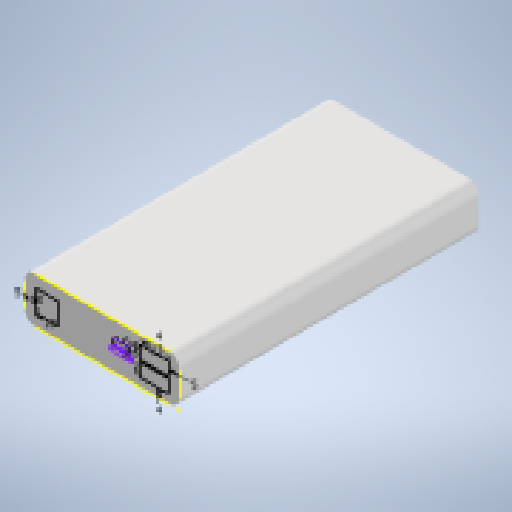
# Autodesk Inventor part: power bank
Saved by Autodesk Inventor 2023 (Build 270158000, 158)
## iProperties
Created: 2023-04-11
Part Number: power bank
Material: Generic
Document SubType Name: Modeling
Designer: ASARe-DAQ-PC
Density: 1 g/cm^3
Appearance: Default
Author: ASARe-DAQ-PC
Autodesk Inventor part; units mm, degrees
ref_plane "YZ Plane" through (0, 0, 0) normal (1, 0, 0) x (0, 1, 0)
ref_plane "XZ Plane" through (0, 0, 0) normal (0, 1, 0) x (-1, 0, 0)
ref_plane "XY Plane" through (0, 0, 0) normal (0, 0, 1) x (1, 0, 0)
sketch "Sketch1" plane through (0, 0, 0) normal (0, 1, 0) x (-1, 0, 0)
  line L0 (0, 0) -> (71, 0)
  line L1 (71, 0) -> (71, -137)
  line L2 (71, -137) -> (0, -137)
  line L3 (0, -137) -> (0, 0)
  dimension "d0" = 137
  dimension "d1" = 71
  constraints: 8 end point, 2 parallel, 1 horizontal, 1 perpendicular
  measures "d0" distance of L2.end L0.start
  measures "d1" distance of L0.start L0.end
extrude "Extrusion1" add sketch "Sketch1" along normal blind 21
fillet "Fillet1" radius 5 4 edges at (0, 21, -68.5) (0, 0, -68.5) (-71, 21, -68.5) (-71, 0, -68.5)
sketch "Sketch2" plane through (-66, 0, 0) normal (0, 0, 1) x (1, 0, 0)
  line L0 (0, 15.5) -> (10, 15.5)
  line L1 (10, 15.5) -> (10, 5.5)
  line L2 (10, 5.5) -> (0, 5.5)
  line L3 (0, 5.5) -> (0, 15.5)
  line L4 (48, 17) -> (61, 17)
  line L5 (61, 17) -> (61, 11)
  line L6 (61, 11) -> (48, 11)
  line L7 (48, 11) -> (48, 17)
  line L8 (48, 10) -> (61, 10)
  line L9 (61, 10) -> (61, 4)
  line L10 (61, 4) -> (48, 4)
  line L11 (48, 4) -> (48, 10)
  line L12 (66, 5) -> (66, 16) projected
  line L13 (0, 0) -> (61, 0) projected
  line L14 (0, 21) -> (61, 21) projected
  line L15 (-5, 5) -> (-5, 16) projected
  line L16 (35.4, 13.6) -> (43, 13.6)
  line L17 (43, 13.6) -> (43, 11)
  line L18 (43, 11) -> (35.4, 11)
  line L19 (35.4, 11) -> (35.4, 13.6)
  line L20 (36.2, 10) -> (42.2, 10)
  line L21 (43.7, 8.5) -> (43.7, 8.3)
  line L22 (42.2, 6.8) -> (36.2, 6.8)
  line L23 (34.7, 8.3) -> (34.7, 8.5)
  arc A0 (36.2, 10) -> (34.7, 8.5) centre (36.2, 8.5) ccw
  arc A1 (43.7, 8.5) -> (42.2, 10) centre (42.2, 8.5) ccw
  arc A2 (34.7, 8.3) -> (36.2, 6.8) centre (36.2, 8.3) ccw
  arc A3 (42.2, 6.8) -> (43.7, 8.3) centre (42.2, 8.3) ccw
  line L24 (35.4, 12) -> (36.4, 11)
  line L25 (43, 12) -> (42, 11)
  point P0 (66, 0)
  point P1 (0, 10.5)
  point P2 (-5, 10.5)
  point P3 (43.7, 6.8)
  point P4 (34.7, 6.8)
  point P5 (39.2, 11)
  point P6 (39.2, 10)
  dimension "d5" = 6
  dimension "d6" = 6
  dimension "d7" = 13
  dimension "d8" = 5
  dimension "d9" = 4
  dimension "d10" = 4
  dimension "d11" = 5
  dimension "d12" = 10
  dimension "d13" = 10
  dimension "d14" = 7.6
  dimension "d15" = 2.6
  dimension "d16" = 5
  dimension "d17" = 3.2
  dimension "d19" = 9
  dimension "d20" = 1
  dimension "d21" = 1.5
  dimension "d26" = 45
  dimension "d27" = 45
  dimension "d28" = 1
  dimension "d29" = 1
  constraints: 44 end point, 10 parallel, 10 point on line, 8 point on circle, 8 tangent, 5 horizontal, 5 perpendicular, 4 centre point, 4 midpoint, 3 equal radius, 2 horizontal alignment, 1 vertical alignment
  measures "d5" distance of L6.end L4.start
  measures "d6" distance of L10.end L8.start
  measures "d7" distance of L4.start L4.end
  measures "d8" distance between parallel lines of L12 L5
  measures "d9" distance between parallel lines of L13 L10
  measures "d10" distance between parallel lines of L14 L4
  measures "d11" distance between parallel lines of L3 L15
  measures "d12" distance of L2.end L0.start
  measures "d13" distance of L1.end L2.end
  measures "d14" distance of L16.start L16.end
  measures "d15" distance of L16.end L17.end
  measures "d16" distance between parallel lines of L7 L17
  measures "d17" distance between parallel lines of L22 L20
  measures "d19" distance of point (43.7, 6.8) point (34.7, 6.8)
  measures "d20" distance between parallel lines of L20 L18
  measures "d21" radius of A0
  measures "d26" angle of L18 L24
  measures "d27" angle of L18 L25
  measures "d28" distance of L18.end L24.start
  measures "d29" distance of L17.end L25.start
extrude "Extrusion2" cut sketch "Sketch2" against normal blind 20 contours L4 L5 L6 L7 | L8 L9 L10 L11 | L16 L17 L25 L18 L24 L19 | L20 A1 L21 A3 L22 A2 L23 A0
extrude "Extrusion3" add sketch "Sketch2" along normal blind 1 contours L0 L1 L2 L3
sketch "Sketch3" plane through (-66, 0, 1) normal (0, 0, 1) x (1, 0, 0)
  circle A0 centre (5, 10.5) radius 3 construction
  arc A1 (3.0716, 12.7981) -> (6.9284, 12.7981) centre (5, 10.5) ccw
  line L0 (3.0716, 12.7981) -> (5, 10.5) construction
  line L1 (5, 10.5) -> (6.9284, 12.7981) construction
  line L2 (5, 10.5) -> (5, 13.5) construction
  line L3 (10, 5.5) -> (10, 15.5) projected
  line L4 (10, 15.5) -> (0, 15.5) projected
  circle A2 centre (5, 10.5) radius 2.5 construction
  arc A3 (3.393, 12.4151) -> (6.607, 12.4151) centre (5, 10.5) ccw
  arc A4 (3.393, 12.4151) -> (3.0716, 12.7981) centre (3.2323, 12.6066) ccw
  arc A5 (6.9284, 12.7981) -> (6.607, 12.4151) centre (6.7677, 12.6066) ccw
  line L5 (4.75, 14) -> (5.25, 14) construction
  line L6 (5.25, 14) -> (5.25, 11.5)
  line L7 (5.25, 11.5) -> (4.75, 11.5) construction
  line L8 (4.75, 11.5) -> (4.75, 14)
  arc A6 (5.25, 14) -> (4.75, 14) centre (5, 14) ccw
  arc A7 (4.75, 11.5) -> (5.25, 11.5) centre (5, 11.5) ccw
  point P0 (66, 0)
  point P1 (10, 10.5)
  point P2 (5, 15.5)
  dimension "d30" = 40
  dimension "d31" = 40
  dimension "d32" = 6
  dimension "d33" = 0.5
  dimension "d34" = 0.5
  dimension "d35" = 2.5
  dimension "d36" = 1
  constraints: 17 point on circle, 14 end point, 8 centre point, 4 midpoint, 3 point on line, 2 coincident, 2 parallel, 2 tangent, 1 concentric, 1 horizontal, 1 horizontal alignment, 1 perpendicular, 1 vertical, 1 vertical alignment
  measures "d30" angle of L2 L0
  measures "d31" angle of L1 L2
  measures "d32" diameter of A0
  measures "d33" radial gap between concentric circles of A0 A2
  measures "d34" distance of L6.end L7.end
  measures "d35" distance of L5.end L6.end
  measures "d36" distance from line of A0.centre L7
extrude "Extrusion4" cut sketch "Sketch3" against normal blind 0.1
body "Solid1"
